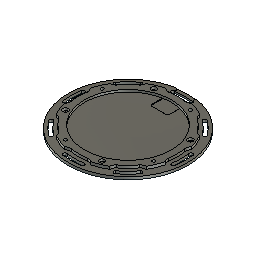
shadowmask_spacer_metallization_fixture (Autodesk Fusion 360 design; units mm, degrees)
Autodesk Fusion 360 part; units mm, degrees
note: some values were not read from the file. Set by a fixed rule: which sketch regions a step uses.
sketch "Sketch1" plane through (0, 0, 0) normal (0, 0, 1) x (1, 0, 0)
  circle A0 centre (0, 0) radius 76.2
  circle A1 centre (0, 0) radius 50
  circle A2 centre (0, 0) radius 67.5
  arc A3 (10.3226, 63.162) -> (-10.3226, 63.162) centre (0, 0) ccw
  arc A4 (9.6774, 59.2144) -> (10.3226, 63.162) centre (10, 61.1882) ccw
  arc A5 (9.6774, 59.2144) -> (-9.6774, 59.2144) centre (0, 0) ccw
  arc A6 (-10.3226, 63.162) -> (-9.6774, 59.2144) centre (-10, 61.1882) ccw
  arc A7 (10, 61.1882) -> (-10, 61.1882) centre (0, 0) ccw construction
  circle A8 centre (20.6649, 49.8895) radius 1.5
  line L0 (0, 0) -> (0, 50)
  line L1 (20.6649, 49.8895) -> (0, 0)
  arc A9 (-36.1955, 50.3377) -> (-50.3377, 36.1955) centre (0, 0) ccw construction
  arc A10 (-35.0279, 48.7139) -> (-48.7139, 35.0279) centre (0, 0) ccw
  arc A11 (-51.9615, 37.3631) -> (-48.7139, 35.0279) centre (-50.3377, 36.1955) ccw
  arc A12 (-35.0279, 48.7139) -> (-37.3631, 51.9615) centre (-36.1955, 50.3377) ccw
  arc A13 (-37.3631, 51.9615) -> (-51.9615, 37.3631) centre (0, 0) ccw
  circle A14 centre (-20.6649, 49.8895) radius 1.5
  arc A15 (-61.1882, 10) -> (-61.1882, -10) centre (0, 0) ccw construction
  arc A16 (-59.2144, 9.6774) -> (-59.2144, -9.6774) centre (0, 0) ccw
  arc A17 (-63.162, -10.3226) -> (-59.2144, -9.6774) centre (-61.1882, -10) ccw
  arc A18 (-59.2144, 9.6774) -> (-63.162, 10.3226) centre (-61.1882, 10) ccw
  arc A19 (-63.162, 10.3226) -> (-63.162, -10.3226) centre (0, 0) ccw
  circle A20 centre (-49.8895, 20.6649) radius 1.5
  arc A21 (-50.3377, -36.1955) -> (-36.1955, -50.3377) centre (0, 0) ccw construction
  arc A22 (-48.7139, -35.0279) -> (-35.0279, -48.7139) centre (0, 0) ccw
  arc A23 (-37.3631, -51.9615) -> (-35.0279, -48.7139) centre (-36.1955, -50.3377) ccw
  arc A24 (-48.7139, -35.0279) -> (-51.9615, -37.3631) centre (-50.3377, -36.1955) ccw
  arc A25 (-51.9615, -37.3631) -> (-37.3631, -51.9615) centre (0, 0) ccw
  circle A26 centre (-49.8895, -20.6649) radius 1.5
  arc A27 (-10, -61.1882) -> (10, -61.1882) centre (0, 0) ccw construction
  arc A28 (-9.6774, -59.2144) -> (9.6774, -59.2144) centre (0, 0) ccw
  arc A29 (10.3226, -63.162) -> (9.6774, -59.2144) centre (10, -61.1882) ccw
  arc A30 (-9.6774, -59.2144) -> (-10.3226, -63.162) centre (-10, -61.1882) ccw
  arc A31 (-10.3226, -63.162) -> (10.3226, -63.162) centre (0, 0) ccw
  circle A32 centre (-20.6649, -49.8895) radius 1.5
  arc A33 (36.1955, -50.3377) -> (50.3377, -36.1955) centre (0, 0) ccw construction
  arc A34 (35.0279, -48.7139) -> (48.7139, -35.0279) centre (0, 0) ccw
  arc A35 (51.9615, -37.3631) -> (48.7139, -35.0279) centre (50.3377, -36.1955) ccw
  arc A36 (35.0279, -48.7139) -> (37.3631, -51.9615) centre (36.1955, -50.3377) ccw
  arc A37 (37.3631, -51.9615) -> (51.9615, -37.3631) centre (0, 0) ccw
  circle A38 centre (20.6649, -49.8895) radius 1.5
  arc A39 (61.1882, -10) -> (61.1882, 10) centre (0, 0) ccw construction
  arc A40 (59.2144, -9.6774) -> (59.2144, 9.6774) centre (0, 0) ccw
  arc A41 (63.162, 10.3226) -> (59.2144, 9.6774) centre (61.1882, 10) ccw
  arc A42 (59.2144, -9.6774) -> (63.162, -10.3226) centre (61.1882, -10) ccw
  arc A43 (63.162, -10.3226) -> (63.162, 10.3226) centre (0, 0) ccw
  circle A44 centre (49.8895, -20.6649) radius 1.5
  arc A45 (50.3377, 36.1955) -> (36.1955, 50.3377) centre (0, 0) ccw construction
  arc A46 (48.7139, 35.0279) -> (35.0279, 48.7139) centre (0, 0) ccw
  arc A47 (37.3631, 51.9615) -> (35.0279, 48.7139) centre (36.1955, 50.3377) ccw
  arc A48 (48.7139, 35.0279) -> (51.9615, 37.3631) centre (50.3377, 36.1955) ccw
  arc A49 (51.9615, 37.3631) -> (37.3631, 51.9615) centre (0, 0) ccw
  circle A50 centre (49.8895, 20.6649) radius 1.5
  dimension "d1" = 152.4
  dimension "d2" = 100
  dimension "d3" = 135
  dimension "d4" = 62
  dimension "d5" = 20
  dimension "d6" = 4
  dimension "d7" = 10
  dimension "d8" = 54
  dimension "d9" = 3
  dimension "d10" = 22.5
  dimension "d12" = 360
  constraint coincident A0.centre A1.centre
  constraint concentric A0 A2
  constraint tangent A3 A4
  constraint tangent A4 A5
  constraint tangent A5 A6
  constraint tangent A3 A6
  constraint coincident A1 L0.end
  constraint vertical L0
  constraint coincident A8.centre L1.start
  measures "d1" diameter of A0
  measures "d2" diameter of A1
  measures "d3" diameter of A2
  measures "d4" radius of A7
  measures "d5" horizontal distance of A6.centre A4.centre
  measures "d6" distance of A3 A5
  measures "d7" horizontal distance of A0.centre A6.centre
  measures "d8" distance of A0.centre A8.centre
  measures "d9" diameter of A8
  measures "d10" angle of L0 L1
extrude "Extrude1" add sketch "Sketch1" along normal blind 3 contours A1 L0 L1 | A1 L0 L1 | A2 makes body 1
sketch "Sketch2" plane through (0, 0, 3) normal (0, 0, 1) x (-1, 0, 0)
  arc A0 (-9.6774, -59.2144) -> (-10.3226, -63.162) centre (-10, -61.1882) ccw
  arc A1 (-9.6774, -59.2144) -> (9.6774, -59.2144) centre (0, 0) ccw
  arc A2 (10.3226, -63.162) -> (9.6774, -59.2144) centre (10, -61.1882) ccw
  arc A3 (-10.3226, -63.162) -> (10.3226, -63.162) centre (0, 0) ccw
  circle A4 centre (20.6649, -49.8895) radius 1.5
  arc A5 (-48.7139, -35.0279) -> (-51.9615, -37.3631) centre (-50.3377, -36.1955) ccw
  arc A6 (-48.7139, -35.0279) -> (-35.0279, -48.7139) centre (0, 0) ccw
  arc A7 (-37.3631, -51.9615) -> (-35.0279, -48.7139) centre (-36.1955, -50.3377) ccw
  arc A8 (-51.9615, -37.3631) -> (-37.3631, -51.9615) centre (0, 0) ccw
  circle A9 centre (-20.6649, 49.8895) radius 1.5
  circle A10 centre (-49.8895, 20.6649) radius 1.5
  arc A11 (35.0279, -48.7139) -> (37.3631, -51.9615) centre (36.1955, -50.3377) ccw
  arc A12 (35.0279, -48.7139) -> (48.7139, -35.0279) centre (0, 0) ccw
  arc A13 (51.9615, -37.3631) -> (48.7139, -35.0279) centre (50.3377, -36.1955) ccw
  arc A14 (37.3631, -51.9615) -> (51.9615, -37.3631) centre (0, 0) ccw
  circle A15 centre (-49.8895, -20.6649) radius 1.5
  circle A16 centre (-20.6649, -49.8895) radius 1.5
  arc A17 (-35.0279, 48.7139) -> (-37.3631, 51.9615) centre (-36.1955, 50.3377) ccw
  arc A18 (-35.0279, 48.7139) -> (-48.7139, 35.0279) centre (0, 0) ccw
  arc A19 (-51.9615, 37.3631) -> (-48.7139, 35.0279) centre (-50.3377, 36.1955) ccw
  arc A20 (-37.3631, 51.9615) -> (-51.9615, 37.3631) centre (0, 0) ccw
  circle A21 centre (49.8895, -20.6649) radius 1.5
  arc A22 (59.2144, -9.6774) -> (63.162, -10.3226) centre (61.1882, -10) ccw
  arc A23 (59.2144, -9.6774) -> (59.2144, 9.6774) centre (0, 0) ccw
  arc A24 (63.162, 10.3226) -> (59.2144, 9.6774) centre (61.1882, 10) ccw
  arc A25 (63.162, -10.3226) -> (63.162, 10.3226) centre (0, 0) ccw
  arc A26 (9.6774, 59.2144) -> (10.3226, 63.162) centre (10, 61.1882) ccw
  arc A27 (9.6774, 59.2144) -> (-9.6774, 59.2144) centre (0, 0) ccw
  arc A28 (-10.3226, 63.162) -> (-9.6774, 59.2144) centre (-10, 61.1882) ccw
  arc A29 (10.3226, 63.162) -> (-10.3226, 63.162) centre (0, 0) ccw
  circle A30 centre (49.8895, 20.6649) radius 1.5
  circle A31 centre (20.6649, 49.8895) radius 1.5
  arc A32 (-59.2144, 9.6774) -> (-63.162, 10.3226) centre (-61.1882, 10) ccw
  arc A33 (-59.2144, 9.6774) -> (-59.2144, -9.6774) centre (0, 0) ccw
  arc A34 (-63.162, -10.3226) -> (-59.2144, -9.6774) centre (-61.1882, -10) ccw
  arc A35 (-63.162, 10.3226) -> (-63.162, -10.3226) centre (0, 0) ccw
  arc A36 (48.7139, 35.0279) -> (51.9615, 37.3631) centre (50.3377, 36.1955) ccw
  arc A37 (48.7139, 35.0279) -> (35.0279, 48.7139) centre (0, 0) ccw
  arc A38 (37.3631, 51.9615) -> (35.0279, 48.7139) centre (36.1955, 50.3377) ccw
  arc A39 (51.9615, 37.3631) -> (37.3631, 51.9615) centre (0, 0) ccw
  circle A40 centre (0, 0) radius 67.5
  circle A41 centre (0, 0) radius 50.5
  line L0 (15.6924, -48) -> (-15.6924, -48)
  dimension "d15" = 101
  dimension "d16" = 48
  constraint coincident A1.centre A3.centre
  constraint coincident A41 L0.start
  constraint coincident A41 L0.end
  constraint horizontal L0
  measures "d15" diameter of A41
  measures "d16" distance of A1.centre L0
extrude "Extrude2" cut sketch "Sketch2" against normal blind 0.2 contours A41 L0 picked at (9.304, -15.2033) bodies 1
sketch "Sketch3" plane through (0, 0, 3) normal (0, 0, 1) x (-1, 0, 0)
  line L0 (15.6924, -48) -> (-15.6924, -48)
  arc A0 (15.6924, -48) -> (-15.6924, -48) centre (0, 0) ccw
  arc A1 (-9.6774, -59.2144) -> (-10.3226, -63.162) centre (-10, -61.1882) ccw
  arc A2 (-9.6774, -59.2144) -> (9.6774, -59.2144) centre (0, 0) ccw
  arc A3 (10.3226, -63.162) -> (9.6774, -59.2144) centre (10, -61.1882) ccw
  arc A4 (-10.3226, -63.162) -> (10.3226, -63.162) centre (0, 0) ccw
  circle A5 centre (20.6649, -49.8895) radius 1.5
  arc A6 (-48.7139, -35.0279) -> (-51.9615, -37.3631) centre (-50.3377, -36.1955) ccw
  arc A7 (-48.7139, -35.0279) -> (-35.0279, -48.7139) centre (0, 0) ccw
  arc A8 (-37.3631, -51.9615) -> (-35.0279, -48.7139) centre (-36.1955, -50.3377) ccw
  arc A9 (-51.9615, -37.3631) -> (-37.3631, -51.9615) centre (0, 0) ccw
  circle A10 centre (-20.6649, 49.8895) radius 1.5
  circle A11 centre (-49.8895, 20.6649) radius 1.5
  arc A12 (35.0279, -48.7139) -> (37.3631, -51.9615) centre (36.1955, -50.3377) ccw
  arc A13 (35.0279, -48.7139) -> (48.7139, -35.0279) centre (0, 0) ccw
  arc A14 (51.9615, -37.3631) -> (48.7139, -35.0279) centre (50.3377, -36.1955) ccw
  arc A15 (37.3631, -51.9615) -> (51.9615, -37.3631) centre (0, 0) ccw
  circle A16 centre (-49.8895, -20.6649) radius 1.5
  circle A17 centre (-20.6649, -49.8895) radius 1.5
  arc A18 (-35.0279, 48.7139) -> (-37.3631, 51.9615) centre (-36.1955, 50.3377) ccw
  arc A19 (-35.0279, 48.7139) -> (-48.7139, 35.0279) centre (0, 0) ccw
  arc A20 (-51.9615, 37.3631) -> (-48.7139, 35.0279) centre (-50.3377, 36.1955) ccw
  arc A21 (-37.3631, 51.9615) -> (-51.9615, 37.3631) centre (0, 0) ccw
  circle A22 centre (49.8895, -20.6649) radius 1.5
  arc A23 (59.2144, -9.6774) -> (63.162, -10.3226) centre (61.1882, -10) ccw
  arc A24 (59.2144, -9.6774) -> (59.2144, 9.6774) centre (0, 0) ccw
  arc A25 (63.162, 10.3226) -> (59.2144, 9.6774) centre (61.1882, 10) ccw
  arc A26 (63.162, -10.3226) -> (63.162, 10.3226) centre (0, 0) ccw
  arc A27 (9.6774, 59.2144) -> (10.3226, 63.162) centre (10, 61.1882) ccw
  arc A28 (9.6774, 59.2144) -> (-9.6774, 59.2144) centre (0, 0) ccw
  arc A29 (-10.3226, 63.162) -> (-9.6774, 59.2144) centre (-10, 61.1882) ccw
  arc A30 (10.3226, 63.162) -> (-10.3226, 63.162) centre (0, 0) ccw
  circle A31 centre (49.8895, 20.6649) radius 1.5
  circle A32 centre (20.6649, 49.8895) radius 1.5
  arc A33 (-59.2144, 9.6774) -> (-63.162, 10.3226) centre (-61.1882, 10) ccw
  arc A34 (-59.2144, 9.6774) -> (-59.2144, -9.6774) centre (0, 0) ccw
  arc A35 (-63.162, -10.3226) -> (-59.2144, -9.6774) centre (-61.1882, -10) ccw
  arc A36 (-63.162, 10.3226) -> (-63.162, -10.3226) centre (0, 0) ccw
  arc A37 (48.7139, 35.0279) -> (51.9615, 37.3631) centre (50.3377, 36.1955) ccw
  arc A38 (48.7139, 35.0279) -> (35.0279, 48.7139) centre (0, 0) ccw
  arc A39 (37.3631, 51.9615) -> (35.0279, 48.7139) centre (36.1955, 50.3377) ccw
  arc A40 (51.9615, 37.3631) -> (37.3631, 51.9615) centre (0, 0) ccw
  circle A41 centre (0, 0) radius 67.5
  line L1 (-10, -35) -> (10, -35)
  line L2 (10, -35) -> (10, -71.093)
  line L3 (10, -71.093) -> (-10, -71.093)
  line L4 (-10, -71.093) -> (-10, -35)
  dimension "d19" = 10
  dimension "d20" = 35
  dimension "d21" = 20
  constraint horizontal L1
  constraint vertical L2
  constraint horizontal L3
  constraint vertical L4
  measures "d19" distance of A0.centre L4
  measures "d20" distance of A0.centre L1
  measures "d21" distance of L2 L4
extrude "Extrude3" cut sketch "Sketch3" against normal blind 1 contours L0 A1 A2 A3 L2 L4 | L0 L1 L2 L4 | A4 A41 L2 L4 bodies 1
fillet "Fillet1" radius 2 2 edges at (10, 35, 2.4) (-10, 35, 2.4) on bodies 1
fillet "Fillet2" radius 2 2 edges at (10, 66.7551, 2.5) (-10, 66.7551, 2.5) on bodies 1
sketch "Sketch4" plane through (0, 0, 3) normal (0, 0, 1) x (-1, 0, 0) in component "top_plate"
  arc A0 (48.7139, 35.0279) -> (51.9615, 37.3631) centre (50.3377, 36.1955) ccw
  arc A1 (48.7139, 35.0279) -> (35.0279, 48.7139) centre (0, 0) ccw
  arc A2 (37.3631, 51.9615) -> (35.0279, 48.7139) centre (36.1955, 50.3377) ccw
  arc A3 (51.9615, 37.3631) -> (37.3631, 51.9615) centre (0, 0) ccw
  arc A4 (-59.2144, 9.6774) -> (-63.162, 10.3226) centre (-61.1882, 10) ccw
  arc A5 (-59.2144, 9.6774) -> (-59.2144, -9.6774) centre (0, 0) ccw
  arc A6 (-63.162, -10.3226) -> (-59.2144, -9.6774) centre (-61.1882, -10) ccw
  arc A7 (-63.162, 10.3226) -> (-63.162, -10.3226) centre (0, 0) ccw
  circle A8 centre (20.6649, 49.8895) radius 1.5
  circle A9 centre (49.8895, 20.6649) radius 1.5
  arc A10 (9.6774, 59.2144) -> (10.3226, 63.162) centre (10, 61.1882) ccw
  arc A11 (9.6774, 59.2144) -> (-9.6774, 59.2144) centre (0, 0) ccw
  arc A12 (-10.3226, 63.162) -> (-9.6774, 59.2144) centre (-10, 61.1882) ccw
  arc A13 (10.3226, 63.162) -> (-10.3226, 63.162) centre (0, 0) ccw
  arc A14 (59.2144, -9.6774) -> (63.162, -10.3226) centre (61.1882, -10) ccw
  arc A15 (59.2144, -9.6774) -> (59.2144, 9.6774) centre (0, 0) ccw
  arc A16 (63.162, 10.3226) -> (59.2144, 9.6774) centre (61.1882, 10) ccw
  arc A17 (63.162, -10.3226) -> (63.162, 10.3226) centre (0, 0) ccw
  circle A18 centre (49.8895, -20.6649) radius 1.5
  arc A19 (-35.0279, 48.7139) -> (-37.3631, 51.9615) centre (-36.1955, 50.3377) ccw
  arc A20 (-35.0279, 48.7139) -> (-48.7139, 35.0279) centre (0, 0) ccw
  arc A21 (-51.9615, 37.3631) -> (-48.7139, 35.0279) centre (-50.3377, 36.1955) ccw
  arc A22 (-37.3631, 51.9615) -> (-51.9615, 37.3631) centre (0, 0) ccw
  circle A23 centre (-20.6649, -49.8895) radius 1.5
  circle A24 centre (-49.8895, -20.6649) radius 1.5
  arc A25 (35.0279, -48.7139) -> (37.3631, -51.9615) centre (36.1955, -50.3377) ccw
  arc A26 (35.0279, -48.7139) -> (48.7139, -35.0279) centre (0, 0) ccw
  arc A27 (51.9615, -37.3631) -> (48.7139, -35.0279) centre (50.3377, -36.1955) ccw
  arc A28 (37.3631, -51.9615) -> (51.9615, -37.3631) centre (0, 0) ccw
  circle A29 centre (-49.8895, 20.6649) radius 1.5
  circle A30 centre (-20.6649, 49.8895) radius 1.5
  arc A31 (-48.7139, -35.0279) -> (-51.9615, -37.3631) centre (-50.3377, -36.1955) ccw
  arc A32 (-48.7139, -35.0279) -> (-35.0279, -48.7139) centre (0, 0) ccw
  arc A33 (-37.3631, -51.9615) -> (-35.0279, -48.7139) centre (-36.1955, -50.3377) ccw
  arc A34 (-51.9615, -37.3631) -> (-37.3631, -51.9615) centre (0, 0) ccw
  circle A35 centre (20.6649, -49.8895) radius 1.5
  arc A36 (10, -64.3914) -> (12.3664, -66.3575) centre (12, -64.3914) ccw
  arc A37 (12.3664, -66.3575) -> (-12.3664, -66.3575) centre (0, 0) ccw
  arc A38 (-12.3664, -66.3575) -> (-10, -64.3914) centre (-12, -64.3914) ccw
  line L0 (-10, -64.3914) -> (-10, -63.2139)
  arc A39 (-10.3226, -63.162) -> (-10, -63.2139) centre (0, 0) ccw
  arc A40 (-10, -59.1882) -> (-10.3226, -63.162) centre (-10, -61.1882) ccw
  line L1 (-10, -59.1882) -> (-10, -48)
  line L2 (-10, -48) -> (-15.6924, -48)
  arc A41 (15.6924, -48) -> (-15.6924, -48) centre (0, 0) ccw
  line L3 (15.6924, -48) -> (10, -48)
  line L4 (10, -48) -> (10, -59.1882)
  arc A42 (10.3226, -63.162) -> (10, -59.1882) centre (10, -61.1882) ccw
  arc A43 (10, -63.2139) -> (10.3226, -63.162) centre (0, 0) ccw
  line L5 (10, -63.2139) -> (10, -64.3914)
  circle A44 centre (0, 0) radius 49
  circle A45 centre (0, 0) radius 59
  arc A46 (-10.9677, -67.1097) -> (10.9677, -67.1097) centre (0, 0) ccw
  arc A47 (-9.0323, -55.2668) -> (-10.9677, -67.1097) centre (-10, -61.1882) ccw
  arc A48 (-9.0323, -55.2668) -> (9.0323, -55.2668) centre (0, 0) ccw
  arc A49 (10.9677, -67.1097) -> (9.0323, -55.2668) centre (10, -61.1882) ccw
  arc A50 (-10, -61.1882) -> (10, -61.1882) centre (0, 0) ccw construction
  arc A51 (32.6928, -45.4663) -> (39.6983, -55.2091) centre (36.1955, -50.3377) ccw
  arc A52 (55.2091, -39.6983) -> (45.4663, -32.6928) centre (50.3377, -36.1955) ccw
  line L6 (38.4605, -52.6027) -> (37.6279, -51.7701)
  arc A53 (39.6983, -55.2091) -> (55.2091, -39.6983) centre (0, 0) ccw
  arc A54 (32.6928, -45.4663) -> (45.4663, -32.6928) centre (0, 0) ccw
  arc A55 (36.1955, -50.3377) -> (50.3377, -36.1955) centre (0, 0) ccw construction
  arc A56 (34.7813, -48.9235) -> (37.3631, -51.9615) centre (36.1955, -50.3377) ccw
  arc A57 (37.3631, -51.9615) -> (37.6279, -51.7701) centre (0, 0) ccw
  arc A58 (38.1775, -55.6662) -> (38.4605, -52.6027) centre (37.0463, -54.0169) ccw
  line L7 (51.7701, -37.6279) -> (52.6027, -38.4605)
  arc A59 (51.7701, -37.6279) -> (51.9615, -37.3631) centre (0, 0) ccw
  arc A60 (51.9615, -37.3631) -> (48.9235, -34.7813) centre (50.3377, -36.1955) ccw
  arc A61 (52.6027, -38.4605) -> (55.6662, -38.1775) centre (54.0169, -37.0463) ccw
  arc A62 (55.2668, -9.0323) -> (67.1097, -10.9677) centre (61.1882, -10) ccw
  arc A63 (67.1097, 10.9677) -> (55.2668, 9.0323) centre (61.1882, 10) ccw
  line L8 (64.3914, -10) -> (63.2139, -10)
  arc A64 (67.1097, -10.9677) -> (67.1097, 10.9677) centre (0, 0) ccw
  arc A65 (55.2668, -9.0323) -> (55.2668, 9.0323) centre (0, 0) ccw
  arc A66 (61.1882, -10) -> (61.1882, 10) centre (0, 0) ccw construction
  arc A67 (59.1882, -10) -> (63.162, -10.3226) centre (61.1882, -10) ccw
  arc A68 (63.162, -10.3226) -> (63.2139, -10) centre (0, 0) ccw
  arc A69 (66.3575, -12.3664) -> (64.3914, -10) centre (64.3914, -12) ccw
  line L9 (63.2139, 10) -> (64.3914, 10)
  arc A70 (63.2139, 10) -> (63.162, 10.3226) centre (0, 0) ccw
  arc A71 (63.162, 10.3226) -> (59.1882, 10) centre (61.1882, 10) ccw
  arc A72 (64.3914, 10) -> (66.3575, 12.3664) centre (64.3914, 12) ccw
  arc A73 (45.4663, 32.6928) -> (55.2091, 39.6983) centre (50.3377, 36.1955) ccw
  arc A74 (39.6983, 55.2091) -> (32.6928, 45.4663) centre (36.1955, 50.3377) ccw
  line L10 (52.6027, 38.4605) -> (51.7701, 37.6279)
  arc A75 (55.2091, 39.6983) -> (39.6983, 55.2091) centre (0, 0) ccw
  arc A76 (45.4663, 32.6928) -> (32.6928, 45.4663) centre (0, 0) ccw
  arc A77 (50.3377, 36.1955) -> (36.1955, 50.3377) centre (0, 0) ccw construction
  arc A78 (48.9235, 34.7813) -> (51.9615, 37.3631) centre (50.3377, 36.1955) ccw
  arc A79 (51.9615, 37.3631) -> (51.7701, 37.6279) centre (0, 0) ccw
  arc A80 (55.6662, 38.1775) -> (52.6027, 38.4605) centre (54.0169, 37.0463) ccw
  line L11 (37.6279, 51.7701) -> (38.4605, 52.6027)
  arc A81 (37.6279, 51.7701) -> (37.3631, 51.9615) centre (0, 0) ccw
  arc A82 (37.3631, 51.9615) -> (34.7813, 48.9235) centre (36.1955, 50.3377) ccw
  arc A83 (38.4605, 52.6027) -> (38.1775, 55.6662) centre (37.0463, 54.0169) ccw
  arc A84 (9.0323, 55.2668) -> (10.9677, 67.1097) centre (10, 61.1882) ccw
  arc A85 (-10.9677, 67.1097) -> (-9.0323, 55.2668) centre (-10, 61.1882) ccw
  line L12 (10, 64.3914) -> (10, 63.2139)
  arc A86 (10.9677, 67.1097) -> (-10.9677, 67.1097) centre (0, 0) ccw
  arc A87 (9.0323, 55.2668) -> (-9.0323, 55.2668) centre (0, 0) ccw
  arc A88 (10, 61.1882) -> (-10, 61.1882) centre (0, 0) ccw construction
  arc A89 (10, 59.1882) -> (10.3226, 63.162) centre (10, 61.1882) ccw
  arc A90 (10.3226, 63.162) -> (10, 63.2139) centre (0, 0) ccw
  arc A91 (12.3664, 66.3575) -> (10, 64.3914) centre (12, 64.3914) ccw
  line L13 (-10, 63.2139) -> (-10, 64.3914)
  arc A92 (-10, 63.2139) -> (-10.3226, 63.162) centre (0, 0) ccw
  arc A93 (-10.3226, 63.162) -> (-10, 59.1882) centre (-10, 61.1882) ccw
  arc A94 (-10, 64.3914) -> (-12.3664, 66.3575) centre (-12, 64.3914) ccw
  arc A95 (-32.6928, 45.4663) -> (-39.6983, 55.2091) centre (-36.1955, 50.3377) ccw
  arc A96 (-55.2091, 39.6983) -> (-45.4663, 32.6928) centre (-50.3377, 36.1955) ccw
  line L14 (-38.4605, 52.6027) -> (-37.6279, 51.7701)
  arc A97 (-39.6983, 55.2091) -> (-55.2091, 39.6983) centre (0, 0) ccw
  arc A98 (-32.6928, 45.4663) -> (-45.4663, 32.6928) centre (0, 0) ccw
  arc A99 (-36.1955, 50.3377) -> (-50.3377, 36.1955) centre (0, 0) ccw construction
  arc A100 (-34.7813, 48.9235) -> (-37.3631, 51.9615) centre (-36.1955, 50.3377) ccw
  arc A101 (-37.3631, 51.9615) -> (-37.6279, 51.7701) centre (0, 0) ccw
  arc A102 (-38.1775, 55.6662) -> (-38.4605, 52.6027) centre (-37.0463, 54.0169) ccw
  line L15 (-51.7701, 37.6279) -> (-52.6027, 38.4605)
  arc A103 (-51.7701, 37.6279) -> (-51.9615, 37.3631) centre (0, 0) ccw
  arc A104 (-51.9615, 37.3631) -> (-48.9235, 34.7813) centre (-50.3377, 36.1955) ccw
  arc A105 (-52.6027, 38.4605) -> (-55.6662, 38.1775) centre (-54.0169, 37.0463) ccw
  arc A106 (-55.2668, 9.0323) -> (-67.1097, 10.9677) centre (-61.1882, 10) ccw
  arc A107 (-67.1097, -10.9677) -> (-55.2668, -9.0323) centre (-61.1882, -10) ccw
  line L16 (-64.3914, 10) -> (-63.2139, 10)
  arc A108 (-67.1097, 10.9677) -> (-67.1097, -10.9677) centre (0, 0) ccw
  arc A109 (-55.2668, 9.0323) -> (-55.2668, -9.0323) centre (0, 0) ccw
  arc A110 (-61.1882, 10) -> (-61.1882, -10) centre (0, 0) ccw construction
  arc A111 (-59.1882, 10) -> (-63.162, 10.3226) centre (-61.1882, 10) ccw
  arc A112 (-63.162, 10.3226) -> (-63.2139, 10) centre (0, 0) ccw
  arc A113 (-66.3575, 12.3664) -> (-64.3914, 10) centre (-64.3914, 12) ccw
  line L17 (-63.2139, -10) -> (-64.3914, -10)
  arc A114 (-63.2139, -10) -> (-63.162, -10.3226) centre (0, 0) ccw
  arc A115 (-63.162, -10.3226) -> (-59.1882, -10) centre (-61.1882, -10) ccw
  arc A116 (-64.3914, -10) -> (-66.3575, -12.3664) centre (-64.3914, -12) ccw
  arc A117 (-45.4663, -32.6928) -> (-55.2091, -39.6983) centre (-50.3377, -36.1955) ccw
  arc A118 (-39.6983, -55.2091) -> (-32.6928, -45.4663) centre (-36.1955, -50.3377) ccw
  line L18 (-52.6027, -38.4605) -> (-51.7701, -37.6279)
  arc A119 (-55.2091, -39.6983) -> (-39.6983, -55.2091) centre (0, 0) ccw
  arc A120 (-45.4663, -32.6928) -> (-32.6928, -45.4663) centre (0, 0) ccw
  arc A121 (-50.3377, -36.1955) -> (-36.1955, -50.3377) centre (0, 0) ccw construction
  arc A122 (-48.9235, -34.7813) -> (-51.9615, -37.3631) centre (-50.3377, -36.1955) ccw
  arc A123 (-51.9615, -37.3631) -> (-51.7701, -37.6279) centre (0, 0) ccw
  arc A124 (-55.6662, -38.1775) -> (-52.6027, -38.4605) centre (-54.0169, -37.0463) ccw
  line L19 (-37.6279, -51.7701) -> (-38.4605, -52.6027)
  arc A125 (-37.6279, -51.7701) -> (-37.3631, -51.9615) centre (0, 0) ccw
  arc A126 (-37.3631, -51.9615) -> (-34.7813, -48.9235) centre (-36.1955, -50.3377) ccw
  arc A127 (-38.4605, -52.6027) -> (-38.1775, -55.6662) centre (-37.0463, -54.0169) ccw
  dimension "d31" = 98
  dimension "d32" = 118
  dimension "d33" = 12
  dimension "d35" = 360
  constraint concentric A1 A44
  constraint concentric A44 A45
  constraint tangent A46 A47
  constraint tangent A47 A48
  constraint tangent A48 A49
  constraint tangent A46 A49
  constraint coincident A1.centre A3.centre
  constraint coincident A40.centre A47.centre
  constraint coincident A42.centre A49.centre
  measures "d31" diameter of A44
  measures "d32" diameter of A45
  measures "d33" distance of A46 A48
extrude "Extrude2'" add sketch "Sketch4" along normal blind 3 separate body contours L1 L2 A41 L3 L4 A45 A47 A49 A51 A52 A54 A62 A63 A65 A73 A74 A76 A84 A85 A87 A95 A96 A98 A106 A107 A109 A117 A118 A120 | L1 L2 A41 L3 L4 A47 A48 A49 makes body 2 in component "top_plate"
sketch "Sketch5" plane through (0, 0, 6) normal (0, 0, 1) x (-1, 0, 0) in component "top_plate"
  circle A0 centre (20.6649, -49.8895) radius 1.5
  circle A1 centre (20.6649, 49.8895) radius 1.5
  circle A2 centre (0, 0) radius 49
  circle A3 centre (-49.8895, 20.6649) radius 1.5
  circle A4 centre (-20.6649, -49.8895) radius 1.5
  circle A5 centre (-20.6649, 49.8895) radius 1.5
  circle A6 centre (-49.8895, -20.6649) radius 1.5
  circle A7 centre (49.8895, 20.6649) radius 1.5
  circle A8 centre (49.8895, -20.6649) radius 1.5
  arc A9 (-57.1958, -14.4789) -> (-50.6817, -30.2054) centre (0, 0) ccw
  arc A10 (-45.4663, -32.6928) -> (-50.6817, -30.2054) centre (-50.3377, -36.1955) ccw
  arc A11 (-45.4663, -32.6928) -> (-32.6928, -45.4663) centre (0, 0) ccw
  arc A12 (-30.2054, -50.6817) -> (-32.6928, -45.4663) centre (-36.1955, -50.3377) ccw
  arc A13 (-30.2054, -50.6817) -> (-14.4789, -57.1958) centre (0, 0) ccw
  arc A14 (-9.0323, -55.2668) -> (-14.4789, -57.1958) centre (-10, -61.1882) ccw
  arc A15 (-9.0323, -55.2668) -> (9.0323, -55.2668) centre (0, 0) ccw
  arc A16 (14.4789, -57.1958) -> (9.0323, -55.2668) centre (10, -61.1882) ccw
  arc A17 (14.4789, -57.1958) -> (30.2054, -50.6817) centre (0, 0) ccw
  arc A18 (32.6928, -45.4663) -> (30.2054, -50.6817) centre (36.1955, -50.3377) ccw
  arc A19 (32.6928, -45.4663) -> (45.4663, -32.6928) centre (0, 0) ccw
  arc A20 (50.6817, -30.2054) -> (45.4663, -32.6928) centre (50.3377, -36.1955) ccw
  arc A21 (50.6817, -30.2054) -> (57.1958, -14.4789) centre (0, 0) ccw
  arc A22 (55.2668, -9.0323) -> (57.1958, -14.4789) centre (61.1882, -10) ccw
  arc A23 (55.2668, -9.0323) -> (55.2668, 9.0323) centre (0, 0) ccw
  arc A24 (57.1958, 14.4789) -> (55.2668, 9.0323) centre (61.1882, 10) ccw
  arc A25 (57.1958, 14.4789) -> (50.6817, 30.2054) centre (0, 0) ccw
  arc A26 (45.4663, 32.6928) -> (50.6817, 30.2054) centre (50.3377, 36.1955) ccw
  arc A27 (45.4663, 32.6928) -> (32.6928, 45.4663) centre (0, 0) ccw
  arc A28 (30.2054, 50.6817) -> (32.6928, 45.4663) centre (36.1955, 50.3377) ccw
  arc A29 (30.2054, 50.6817) -> (14.4789, 57.1958) centre (0, 0) ccw
  arc A30 (9.0323, 55.2668) -> (14.4789, 57.1958) centre (10, 61.1882) ccw
  arc A31 (9.0323, 55.2668) -> (-9.0323, 55.2668) centre (0, 0) ccw
  arc A32 (-14.4789, 57.1958) -> (-9.0323, 55.2668) centre (-10, 61.1882) ccw
  arc A33 (-14.4789, 57.1958) -> (-30.2054, 50.6817) centre (0, 0) ccw
  arc A34 (-32.6928, 45.4663) -> (-30.2054, 50.6817) centre (-36.1955, 50.3377) ccw
  arc A35 (-32.6928, 45.4663) -> (-45.4663, 32.6928) centre (0, 0) ccw
  arc A36 (-50.6817, 30.2054) -> (-45.4663, 32.6928) centre (-50.3377, 36.1955) ccw
  arc A37 (-50.6817, 30.2054) -> (-57.1958, 14.4789) centre (0, 0) ccw
  arc A38 (-55.2668, 9.0323) -> (-57.1958, 14.4789) centre (-61.1882, 10) ccw
  arc A39 (-55.2668, 9.0323) -> (-55.2668, -9.0323) centre (0, 0) ccw
  arc A40 (-57.1958, -14.4789) -> (-55.2668, -9.0323) centre (-61.1882, -10) ccw
  circle A41 centre (20.6649, -49.8895) radius 3
  circle A42 centre (49.8895, 20.6649) radius 3
  circle A43 centre (-20.6649, 49.8895) radius 3
  circle A44 centre (-49.8895, -20.6649) radius 3
  circle A45 centre (49.8895, -20.6649) radius 1.7
  circle A46 centre (20.6649, 49.8895) radius 1.7
  circle A47 centre (-49.8895, 20.6649) radius 1.7
  circle A48 centre (-20.6649, -49.8895) radius 1.7
  dimension "d38" = 6
  dimension "d40" = 360
  dimension "d52" = 3.4
  dimension "d54" = 360
  constraint concentric A0 A41
  constraint concentric A8 A45
  measures "d38" diameter of A41
  measures "d52" diameter of A45
extrude "Extrude3'" cut sketch "Sketch5" against normal blind 3 contours A41 | A42 | A43 | A44 bodies 2 in component "top_plate"
sketch "Sketch7" plane through (0, 0, 0) normal (0, 0, -1) x (1, 0, 0) in component "top_plate"
  arc A0 (10.3226, -63.162) -> (9.6774, -59.2144) centre (10, -61.1882) ccw
  arc A1 (-10.3226, -63.162) -> (10.3226, -63.162) centre (0, 0) ccw
  arc A2 (-9.6774, -59.2144) -> (-10.3226, -63.162) centre (-10, -61.1882) ccw
  arc A3 (-9.6774, -59.2144) -> (9.6774, -59.2144) centre (0, 0) ccw
  circle A4 centre (-20.6649, -49.8895) radius 1.5
  arc A5 (51.9615, -37.3631) -> (48.7139, -35.0279) centre (50.3377, -36.1955) ccw
  arc A6 (37.3631, -51.9615) -> (51.9615, -37.3631) centre (0, 0) ccw
  arc A7 (35.0279, -48.7139) -> (37.3631, -51.9615) centre (36.1955, -50.3377) ccw
  arc A8 (35.0279, -48.7139) -> (48.7139, -35.0279) centre (0, 0) ccw
  circle A9 centre (20.6649, 49.8895) radius 1.5
  circle A10 centre (49.8895, 20.6649) radius 1.5
  arc A11 (-37.3631, -51.9615) -> (-35.0279, -48.7139) centre (-36.1955, -50.3377) ccw
  arc A12 (-51.9615, -37.3631) -> (-37.3631, -51.9615) centre (0, 0) ccw
  arc A13 (-48.7139, -35.0279) -> (-51.9615, -37.3631) centre (-50.3377, -36.1955) ccw
  arc A14 (-48.7139, -35.0279) -> (-35.0279, -48.7139) centre (0, 0) ccw
  circle A15 centre (49.8895, -20.6649) radius 1.5
  circle A16 centre (20.6649, -49.8895) radius 1.5
  arc A17 (37.3631, 51.9615) -> (35.0279, 48.7139) centre (36.1955, 50.3377) ccw
  arc A18 (51.9615, 37.3631) -> (37.3631, 51.9615) centre (0, 0) ccw
  arc A19 (48.7139, 35.0279) -> (51.9615, 37.3631) centre (50.3377, 36.1955) ccw
  arc A20 (48.7139, 35.0279) -> (35.0279, 48.7139) centre (0, 0) ccw
  circle A21 centre (-49.8895, -20.6649) radius 1.5
  arc A22 (-63.162, -10.3226) -> (-59.2144, -9.6774) centre (-61.1882, -10) ccw
  arc A23 (-63.162, 10.3226) -> (-63.162, -10.3226) centre (0, 0) ccw
  arc A24 (-59.2144, 9.6774) -> (-63.162, 10.3226) centre (-61.1882, 10) ccw
  arc A25 (-59.2144, 9.6774) -> (-59.2144, -9.6774) centre (0, 0) ccw
  arc A26 (-10.3226, 63.162) -> (-9.6774, 59.2144) centre (-10, 61.1882) ccw
  arc A27 (10.3226, 63.162) -> (-10.3226, 63.162) centre (0, 0) ccw
  arc A28 (9.6774, 59.2144) -> (10.3226, 63.162) centre (10, 61.1882) ccw
  arc A29 (9.6774, 59.2144) -> (-9.6774, 59.2144) centre (0, 0) ccw
  circle A30 centre (-49.8895, 20.6649) radius 1.5
  circle A31 centre (-20.6649, 49.8895) radius 1.5
  arc A32 (63.162, 10.3226) -> (59.2144, 9.6774) centre (61.1882, 10) ccw
  arc A33 (63.162, -10.3226) -> (63.162, 10.3226) centre (0, 0) ccw
  arc A34 (59.2144, -9.6774) -> (63.162, -10.3226) centre (61.1882, -10) ccw
  arc A35 (59.2144, -9.6774) -> (59.2144, 9.6774) centre (0, 0) ccw
  arc A36 (-51.9615, 37.3631) -> (-48.7139, 35.0279) centre (-50.3377, 36.1955) ccw
  arc A37 (-37.3631, 51.9615) -> (-51.9615, 37.3631) centre (0, 0) ccw
  arc A38 (-35.0279, 48.7139) -> (-37.3631, 51.9615) centre (-36.1955, 50.3377) ccw
  arc A39 (-35.0279, 48.7139) -> (-48.7139, 35.0279) centre (0, 0) ccw
  circle A40 centre (0, 0) radius 67.5
sketch "Sketch8" plane through (0, 0, 3) normal (0, 0, -1) x (1, 0, 0) in component "top_plate"
  circle A0 centre (49.8895, -20.6649) radius 3
  circle A1 centre (-49.8895, 20.6649) radius 3
  circle A2 centre (-20.6649, -49.8895) radius 3
  circle A3 centre (20.6649, 49.8895) radius 3
  circle A4 centre (-20.6649, 49.8895) radius 1.5
  circle A5 centre (0, 0) radius 49
  circle A6 centre (49.8895, 20.6649) radius 1.5
  circle A7 centre (20.6649, -49.8895) radius 1.5
  circle A8 centre (-49.8895, -20.6649) radius 1.5
  arc A9 (50.6817, -30.2054) -> (57.1958, -14.4789) centre (0, 0) ccw
  arc A10 (55.2668, -9.0323) -> (57.1958, -14.4789) centre (61.1882, -10) ccw
  arc A11 (55.2668, -9.0323) -> (55.2668, 9.0323) centre (0, 0) ccw
  arc A12 (57.1958, 14.4789) -> (55.2668, 9.0323) centre (61.1882, 10) ccw
  arc A13 (57.1958, 14.4789) -> (50.6817, 30.2054) centre (0, 0) ccw
  arc A14 (45.4663, 32.6928) -> (50.6817, 30.2054) centre (50.3377, 36.1955) ccw
  arc A15 (45.4663, 32.6928) -> (32.6928, 45.4663) centre (0, 0) ccw
  arc A16 (30.2054, 50.6817) -> (32.6928, 45.4663) centre (36.1955, 50.3377) ccw
  arc A17 (30.2054, 50.6817) -> (14.4789, 57.1958) centre (0, 0) ccw
  arc A18 (9.0323, 55.2668) -> (14.4789, 57.1958) centre (10, 61.1882) ccw
  arc A19 (9.0323, 55.2668) -> (-9.0323, 55.2668) centre (0, 0) ccw
  arc A20 (-14.4789, 57.1958) -> (-9.0323, 55.2668) centre (-10, 61.1882) ccw
  arc A21 (-14.4789, 57.1958) -> (-30.2054, 50.6817) centre (0, 0) ccw
  arc A22 (-32.6928, 45.4663) -> (-30.2054, 50.6817) centre (-36.1955, 50.3377) ccw
  arc A23 (-32.6928, 45.4663) -> (-45.4663, 32.6928) centre (0, 0) ccw
  arc A24 (-50.6817, 30.2054) -> (-45.4663, 32.6928) centre (-50.3377, 36.1955) ccw
  arc A25 (-50.6817, 30.2054) -> (-57.1958, 14.4789) centre (0, 0) ccw
  arc A26 (-55.2668, 9.0323) -> (-57.1958, 14.4789) centre (-61.1882, 10) ccw
  arc A27 (-55.2668, 9.0323) -> (-55.2668, -9.0323) centre (0, 0) ccw
  arc A28 (-57.1958, -14.4789) -> (-55.2668, -9.0323) centre (-61.1882, -10) ccw
  arc A29 (-57.1958, -14.4789) -> (-50.6817, -30.2054) centre (0, 0) ccw
  arc A30 (-45.4663, -32.6928) -> (-50.6817, -30.2054) centre (-50.3377, -36.1955) ccw
  arc A31 (-45.4663, -32.6928) -> (-32.6928, -45.4663) centre (0, 0) ccw
  arc A32 (-30.2054, -50.6817) -> (-32.6928, -45.4663) centre (-36.1955, -50.3377) ccw
  arc A33 (-30.2054, -50.6817) -> (-14.4789, -57.1958) centre (0, 0) ccw
  arc A34 (-9.0323, -55.2668) -> (-14.4789, -57.1958) centre (-10, -61.1882) ccw
  arc A35 (-9.0323, -55.2668) -> (9.0323, -55.2668) centre (0, 0) ccw
  arc A36 (14.4789, -57.1958) -> (9.0323, -55.2668) centre (10, -61.1882) ccw
  arc A37 (14.4789, -57.1958) -> (30.2054, -50.6817) centre (0, 0) ccw
  arc A38 (32.6928, -45.4663) -> (30.2054, -50.6817) centre (36.1955, -50.3377) ccw
  arc A39 (32.6928, -45.4663) -> (45.4663, -32.6928) centre (0, 0) ccw
  arc A40 (50.6817, -30.2054) -> (45.4663, -32.6928) centre (50.3377, -36.1955) ccw
  circle A41 centre (0, 0) radius 54
  constraint concentric A5 A41
  constraint coincident A4.centre A41
extrude "Extrude5" cut sketch "Sketch8" against normal blind 0.5 contours A0 A1 A2 A3 A4 A6 A7 A8 A41 bodies 2 in component "top_plate"
fillet "Fillet1'" radius 2 16 edges at (50.9601, 17.8624, 3.25) (48.6649, 23.4036, 3.25) (22.0426, 49.2963, 3.25) (19.2712, 50.4442, 3.25) (-17.8624, 50.9601, 3.25) (-23.4036, 48.6649, 3.25) (-49.2963, 22.0426, 3.25) (-50.4442, 19.2712, 3.25) (-48.6649, -23.4036, 3.25) (-50.9601, -17.8624, 3.25) (-19.2712, -50.4442, 3.25) (-22.0426, -49.2963, 3.25) (23.4036, -48.6649, 3.25) (17.8624, -50.9601, 3.25) (50.4442, -19.2712, 3.25) (49.2963, -22.0426, 3.25) on bodies 2 in component "top_plate"
extrude "Extrude6" cut sketch "Sketch5" against normal blind 3 contours A45 | A46 | A47 | A48 bodies 2 in component "top_plate"
copy_body "Body->Comp1" bodies 1 removing the originals makes body 3 in component "4in_wafer_baseplate"
component "top_plate" placed x (1, 0, 0) y (0, 1, 0) z (0, 0, 1) at (0, 0, 0)
component "4in_wafer_baseplate" placed x (1, 0, 0) y (0, 1, 0) z (0, 0, 1) at (0, 0, 0)
